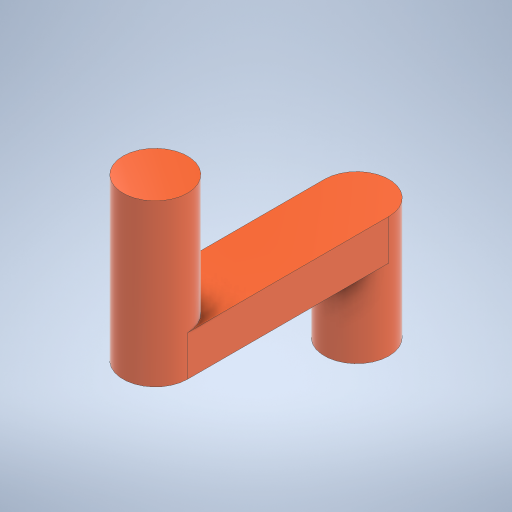
# Autodesk Inventor part: Vevarm
Saved by Autodesk Inventor 2024 (Build 280153020, 153B)
## iProperties
Created: 2023-09-25
Part Number: Vevarm
Material: Generic
Document SubType Name: Modeling
Designer: 23also
Density: 1 g/cm^3
Appearance: Default
Author: 23also
Autodesk Inventor part; units mm, degrees
ref_plane "YZ Plane" through (0, 0, 0) normal (1, 0, 0) x (0, 1, 0)
ref_plane "XZ Plane" through (0, 0, 0) normal (0, 1, 0) x (-1, 0, 0)
ref_plane "XY Plane" through (0, 0, 0) normal (0, 0, 1) x (1, 0, 0)
sketch "Sketch1" plane through (0, 0, 0) normal (0, 1, 0) x (-1, 0, 0)
  circle A0 centre (0, 0) radius 4
  dimension "d0" = 8
  constraints: 1 centre point, 1 coincident
  measures "d0" diameter of A0
extrude "Extrusion1" add sketch "Sketch1" along normal blind 10
sketch "Sketch2" plane through (0, 10, 0) normal (0, 1, 0) x (1, 0, 0)
  circle A0 centre (0, 0) radius 4
  line L0 (4, 0) -> (-4, 0)
  line L1 (-4, 0) -> (-4, -25)
  line L2 (-4, -25) -> (4, -25)
  line L3 (4, -25) -> (4, 0)
  circle A1 centre (0, -25) radius 4
  dimension "d3" = 25
  constraints: 8 end point, 2 parallel, 1 coincident, 1 horizontal, 1 midpoint, 1 perpendicular, 6 other
  measures "d3" distance of L1.end L0.end
extrude "Extrusion2" add sketch "Sketch2" along normal blind 5
sketch "Sketch3" plane through (0, 15, 0) normal (0, 1, 0) x (1, 0, 0)
  arc A0 (-4, -25) -> (4, -25) centre (0, -25) ccw projected
  circle A1 centre (0, -25) radius 4
  point P0 (0, 0)
  constraints: 1 coincident, 3 other
extrude "Extrusion3" add sketch "Sketch3" along normal blind 15
body "Solid1"
